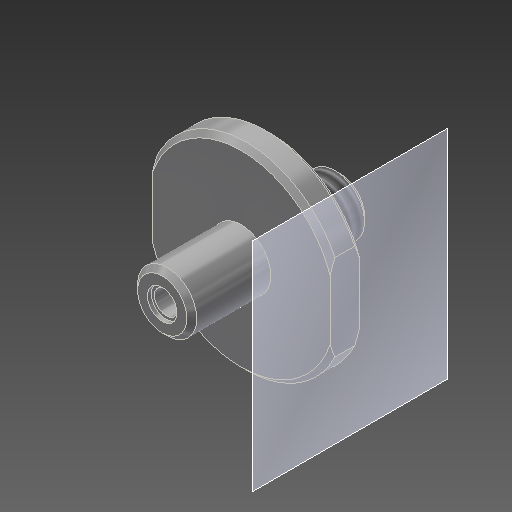
# Autodesk Inventor part: 07
Saved by Autodesk Inventor 2021.1 (Build 251245010, 245A)
## iProperties
Created: 2008-11-14
Part Number: 07
Document SubType Name: Modeling
Density: 8.08 g/cm^3
Material: SUS303
Mass: 9.97845 g
Surface Area: 11.5694 cm^2
Volume: 1.23496 cm^3
Appearance: 鋼
個数: 1
尺度: 2:1
Title: 吸着ブロック
Autodesk Inventor part; units mm, degrees
ref_plane "XZ Plane" through (0, 0, 0) normal (0, 1, 0) x (-1, 0, 0)
ref_plane "XY Plane" through (0, 0, 0) normal (0, 0, 1) x (1, 0, 0)
sketch "スケッチ1" plane through (0, 0, 0) normal (0, 0, 1) x (1, 0, 0)
  circle A0 centre (0, 0) radius 10
  dimension "d0" = 20
  constraints: 1 centre point, 1 coincident
  measures "d0" diameter of A0
extrude "押し出し1" add sketch "スケッチ1" along normal blind 3
sketch "スケッチ2" plane through (0, 0, 3) normal (0, 0, 1) x (1, 0, 0)
  circle A0 centre (0, 0) radius 10 projected
  circle A1 centre (0, 0) radius 3
  dimension "d3" = 6
  constraints: 1 centre point, 1 coincident
  measures "d3" diameter of A1
extrude "押し出し2" add sketch "スケッチ2" along normal blind 8 contours A1
sketch "スケッチ3" plane through (0, 0, 11) normal (0, 0, 1) x (1, 0, 0)
  circle A0 centre (0, 0) radius 3 projected
hole "穴1" at (0, 0, 11) direction (0, 0, -1) diameter 3 depth 0.4
sketch "スケッチ4" plane through (0, 0, 10.6) normal (0, 0, 1) x (1, 0, 0)
  circle A0 centre (0, 0) radius 1.5 projected
hole "穴2" at (0, 0, 10.6) direction (0, 0, -1) diameter 2.4 depth 1.6
sketch "スケッチ5" plane through (0, 0, 9) normal (0, 0, 1) x (1, 0, 0)
  circle A0 centre (0, 0) radius 1.2 projected
hole "穴3" at (0, 0, 9) direction (0, 0, -1) diameter 1.2 end through all
sketch "スケッチ6" plane through (0, 0, 0) normal (0, 0, -1) x (-1, 0, 0)
  circle A0 centre (0, 0) radius 0.6 projected
hole "穴4" at (0, 0, 0) direction (0, 0, 1) diameter 2 depth 6
sketch "スケッチ7" plane through (0, 0, 0) normal (0, 0, -1) x (-1, 0, 0)
  circle A0 centre (0, 0) radius 1 projected
  circle A1 centre (0, 0) radius 10 projected
  circle A2 centre (0, 0) radius 2.2
  dimension "d34" = 4.4
  constraints: 1 centre point, 1 coincident
  measures "d34" diameter of A2
extrude "押し出し3" add sketch "スケッチ7" along normal blind 2 contours A2
sketch "スケッチ8" plane through (0, 0, -2) normal (0, 0, -1) x (-1, 0, 0)
  circle A0 centre (0, 0) radius 1 projected
  circle A1 centre (0, 0) radius 2.2 projected
  circle A2 centre (0, 0) radius 3
  dimension "d39" = 6
  constraints: 1 centre point, 1 coincident
  measures "d39" diameter of A2
extrude "押し出し4" add sketch "スケッチ8" along normal blind 5 contours A1 | A2
thread "ねじ2" size "M6x1" class "6g" standard "ANSI Metric M Profile" length 10
chamfer "面取り1" distance 0.5 angle 45 4 edges at (3, 0, -7) (-10, 0, 0) (-10, 0, 3) (-3, 0, 11)
ref_plane "作業平面1" through (10, 0, 0) normal (1, 0, 0) x (0, 1, 0)
sketch "スケッチ9" plane through (10, 0, 0) normal (1, 0, 0) x (0, 1, 0)
  line L0 (-12.6866, 6.4054) -> (12.2994, 6.4054)
  line L1 (12.2994, 6.4054) -> (12.2994, -2.1864)
  line L2 (12.2994, -2.1864) -> (-12.6866, -2.1864)
  line L3 (-12.6866, -2.1864) -> (-12.6866, 6.4054)
  point P0 (0, 0)
  constraints: 8 end point, 2 parallel, 1 horizontal, 1 perpendicular
extrude "押し出し5" cut sketch "スケッチ9" against normal blind 1
mirror "ミラー1" about plane through (0, 0, 0) normal (1, 0, 0) of "押し出し5"
